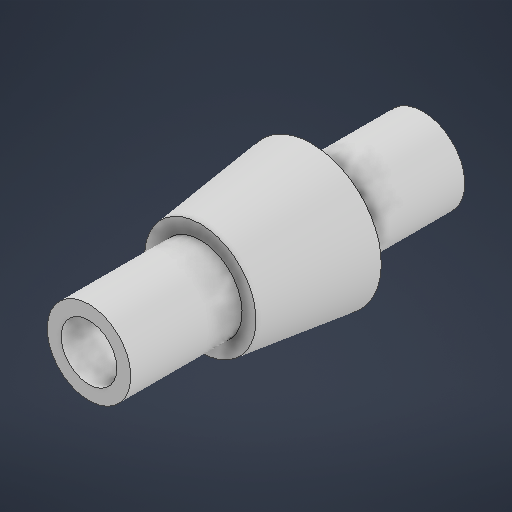
# Autodesk Inventor part: Part3
Saved by Autodesk Inventor 2026 (Build 300175050, 175E)
## iProperties
Created: 2026-04-09
Part Number: Part3
Material: Generic
Document SubType Name: Modeling
Designer: Administrator
Density: 1 g/cm^3
Appearance: Default
Author: Administrator
Autodesk Inventor part; units mm, degrees
ref_plane "YZ Plane" through (0, 0, 0) normal (1, 0, 0) x (0, 1, 0)
ref_plane "XZ Plane" through (0, 0, 0) normal (0, 1, 0) x (-1, 0, 0)
ref_plane "XY Plane" through (0, 0, 0) normal (0, 0, 1) x (1, 0, 0)
sketch "Sketch1" plane through (0, 0, 0) normal (1, 0, 0) x (0, 1, 0)
  line L0 (0, 0) -> (0, -60)
  line L1 (0, -60) -> (7.5, -60)
  line L2 (7.5, -60) -> (7.5, -40)
  line L3 (7.5, -40) -> (12.5, -40)
  line L4 (12.5, -40) -> (10, -20)
  line L5 (10, -20) -> (7.5, -20)
  line L6 (7.5, -20) -> (7.5, 0)
  line L7 (7.5, 0) -> (0, 0)
  dimension "d0" = 40
  dimension "d1" = 20
  dimension "d2" = 2.5
  dimension "d3" = 5
  dimension "d4" = 15
  dimension "d5" = 20
  constraints: 16 end point, 4 perpendicular, 2 vertical, 1 parallel, 1 point on line
  measures "d0" distance between parallel lines of L1 L5
  measures "d1" distance between parallel lines of L1 L3
  measures "d2" distance of L4.end L5.end
  measures "d3" distance of L2.end L3.end
  measures "d4" diameter of L6 L0
  measures "d5" distance between parallel lines of L7 L5
revolve "Revolution1" add sketch "Sketch1" angle 360 about axis through (0, 0, 0) along (0, 0, -1)
sketch "Sketch2" plane through (0, 0, 0) normal (0, 0, 1) x (1, 0, 0)
  circle A0 centre (0, 0) radius 5
  dimension "d10" = 10
  constraints: 1 centre point, 1 coincident
  measures "d10" diameter of A0
extrude "Extrusion2" cut sketch "Sketch2" against normal through all
body "Solid1"
